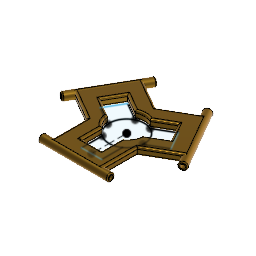
Efector Final v2 (Autodesk Fusion 360 design; units mm, degrees)
Autodesk Fusion 360 part; units mm, degrees
note: some values were not read from the file. Chosen so that the rebuilt part matches the saved one: which pieces of a blend or face edit are solid. Set by a fixed rule: which sketch regions a step uses.
sketch "Boceto1" plane through (0, 0, 0) normal (0, 0, 1) x (1, 0, 0)
  line L0 (-0.0091, 100) -> (-86.598, -50.0079)
  line L1 (-86.598, -50.0079) -> (86.6071, -49.9921)
  line L2 (86.6071, -49.9921) -> (-0.0091, 100)
  circle A0 centre (0, 0) radius 50
  line L3 (-25, 0) -> (25, 0)
  line L4 (-25, 0) -> (-24.9954, -50.0023)
  line L5 (25, 0) -> (25.0046, -49.9977)
  line L6 (12.5, -21.6506) -> (55.801, 3.3545)
  line L7 (12.5, -21.6506) -> (-12.5, 21.6506)
  line L8 (-12.5, 21.6506) -> (30.797, 46.6535)
  line L9 (12.5, 21.6506) -> (-30.8055, 46.6478)
  line L10 (12.5, 21.6506) -> (-12.5, -21.6506)
  line L11 (-12.5, -21.6506) -> (-55.8016, 3.3443)
  dimension "d3" = 50
  dimension "d4" = 50
  dimension "d6" = 360
  constraint coincident A0.centre origin
  constraint tangent L2 A0
  constraint horizontal L3
  constraint midpoint A0.centre L3
  constraint coincident L1 L4.end
  constraint perpendicular L1 L4
  constraint coincident L1 L5.end
  constraint perpendicular L1 L5
  measures "d3" distance of A0.centre L2
  measures "d4" distance of L3.start L3.end
extrude "Extruir1" add sketch "Boceto1" along normal blind 8 contours L0 A0 L9 | L2 A0 L8 | L0 A0 L11 | A0 L3 L4 L7 L8 L9 L11 | L2 A0 L6 | A0 L3 L5 L6 L8 L9 L10 | L7 L8 L9 L10 | A0 L4 L5 L6 L7 L10 L11 | L1 A0 L4 | L3 L4 L10 L11 | L3 L5 L6 L7 | L1 A0 L5 makes body 1
sketch "Boceto2" plane through (-12.498, -21.6518, 0) normal (-0.499921, -0.866071, 0) x (0.866071, -0.499921, 0)
  line L0 (-50, 0) -> (-14.4338, 0)
  line L1 (-14.4338, 0) -> (-14.4338, 8)
  line L2 (-14.4338, 8) -> (-50, 8)
  line L3 (-50, 8) -> (-50, 0)
  circle A0 centre (-50, 4) radius 2
  circle A1 centre (-50, 4) radius 4
  dimension "d9" = 4
  dimension "d10" = 8
  constraint midpoint L3 A0.centre
  constraint concentric A0 A1
  measures "d9" diameter of A0
  measures "d10" diameter of A1
extrude "Extruir2" add sketch "Boceto2" along normal blind 9.5 and the other way blind 59.5 separate body contours L3 A0 A1 | L3 A0 A1 makes body 2
sketch "Boceto3" plane through (17.2473, 29.8795, 0) normal (0.499921, 0.866071, 0) x (-0.866071, 0.499921, 0)
  circle A0 centre (50, 4) radius 2
  circle A1 centre (50, 4) radius 4
extrude "Extruir3" cut sketch "Boceto3" along normal mid plane 348 contours A0 bodies 1
sketch "Boceto4" plane through (-12.502, 21.6495, 0) normal (-0.500079, 0.86598, 0) x (-0.86598, -0.500079, 0)
  line L0 (-50, 0) -> (-14.4338, 0)
  line L1 (-14.4338, 0) -> (-14.4338, 8)
  line L2 (-14.4338, 8) -> (-50, 8)
  line L3 (-50, 8) -> (-50, 0)
  circle A0 centre (-50, 4) radius 2
  circle A1 centre (-50, 4) radius 4
  dimension "d17" = 4
  dimension "d18" = 8
  constraint midpoint L3 A0.centre
  constraint concentric A0 A1
  measures "d17" diameter of A0
  measures "d18" diameter of A1
extrude "Extruir4" add sketch "Boceto4" along normal blind 9.5 and the other way blind 59.5 separate body contours L3 A0 A1 | L3 A0 A1 makes body 3
sketch "Boceto5" plane through (-17.2527, 29.8763, 0) normal (-0.500079, 0.86598, 0) x (-0.86598, -0.500079, 0)
  circle A0 centre (-50, 4) radius 2
  circle A1 centre (-50, 4) radius 4
extrude "Extruir5" cut sketch "Boceto5" along normal mid plane 532 contours A0 bodies 1
sketch "Boceto6" plane through (-25, -0.0023, 0) normal (-1, -0.000091, 0) x (0.000091, -1, 0)
  line L0 (14.4338, 0) -> (50, 0)
  line L1 (50, 0) -> (50, 8)
  line L2 (50, 8) -> (14.4338, 8)
  line L3 (14.4338, 8) -> (14.4338, 0)
  circle A0 centre (50, 4) radius 2
  circle A1 centre (50, 4) radius 4
  dimension "d25" = 4
  dimension "d26" = 8
  constraint midpoint L1 A0.centre
  constraint concentric A0 A1
  measures "d25" diameter of A0
  measures "d26" diameter of A1
extrude "Extruir6" add sketch "Boceto6" along normal blind 9.5 and the other way blind 59.5 separate body contours L1 A0 A1 | L1 A0 A1 makes body 4
sketch "Boceto7" plane through (-34.5, -0.0032, 0) normal (-1, -0.000091, 0) x (0.000091, -1, 0)
  circle A0 centre (50, 4) radius 2
  circle A1 centre (50, 4) radius 4
extrude "Extruir7" cut sketch "Boceto7" along normal mid plane 216 contours A0 bodies 1
sketch "Boceto8" plane through (0, 0, 0) normal (0, 0, 1) x (1, 0, 0)
  circle A0 centre (0, 0) radius 17.5
  line L0 (0, 0) -> (0, -35) construction
  line L1 (10, -35) -> (10, -14.3614)
  line L2 (-10, -35) -> (-10, -14.3614)
  line L3 (-10, -35) -> (10, -35)
  line L4 (25.3109, 26.1603) -> (7.4373, 15.841)
  line L5 (35.3109, 8.8397) -> (25.3109, 26.1603)
  line L6 (35.3109, 8.8397) -> (17.4373, -1.4796)
  line L7 (-35.3109, 8.8397) -> (-17.4373, -1.4796)
  line L8 (-25.3109, 26.1603) -> (-35.3109, 8.8397)
  line L9 (-25.3109, 26.1603) -> (-7.4373, 15.841)
  dimension "d33" = 35
  dimension "d34" = 35
  dimension "d36" = 20
  dimension "d38" = 360
  constraint coincident A0.centre L0.start
  constraint vertical L0
  constraint coincident A0 L1.end
  constraint symmetric L0 L1.start L2.start
  constraint symmetric L0 L1.end L2.end
  constraint perpendicular L1 L3
  measures "d33" diameter of A0
  measures "d34" distance of A0.centre L0.end
  measures "d36" distance of L1.start L2.start
extrude "Extruir8" cut sketch "Boceto8" along normal mid plane 70 bodies 1
extrude "Extruir9" cut sketch "Boceto8" along normal blind 50 bodies 1
fillet "Empalme1" radius 2 tangency weight 2 18 edges at (40.4011, -5.5385, 8) (25.0029, -32.2146, 8) (-24.9971, -32.2192, 8) (-40.4001, -5.5459, 8) (-15.4041, 37.7577, 8) (15.3972, 37.7605, 8) (30.3109, 17.5, 8) (26.3741, 3.6801, 8) (15.1554, -8.75, 8) (10, -24.6807, 8) (0, -35, 8) (-10, -24.6807, 8) (-15.1554, -8.75, 8) (-26.3741, 3.6801, 8) (-30.3109, 17.5, 8) (-16.3741, 21.0006, 8) (0, 17.5, 8) (16.3741, 21.0006, 8) on bodies 1
fillet "Empalme2" radius 2 18 edges at (10, -24.6807, 0) (0, -35, 0) (-10, -24.6807, 0) (15.1554, -8.75, 0) (26.3741, 3.6801, 0) (30.3109, 17.5, 0) (16.3741, 21.0006, 0) (0, 17.5, 0) (-16.3741, 21.0006, 0) (-30.3109, 17.5, 0) (-26.3741, 3.6801, 0) (-15.1554, -8.75, 0) (25.0029, -32.2146, 0) (-24.9971, -32.2192, 0) (40.4011, -5.5385, 0) (15.3972, 37.7605, 0) (-15.4041, 37.7577, 0) (-40.4001, -5.5459, 0) on bodies 1
fillet "Empalme3" radius 1 1 edges at (-34.4958, -46.2738, 2.5535) on bodies 4
fillet "Empalme4" radius 1 5 edges at (-63.7807, -3.0191, 2.5535) (-29.2861, 56.7399, 5.4465) (63.7812, -3.0074, 5.4465) (29.2758, 56.7452, 2.5535) (34.5042, -46.2675, 5.4465) on bodies 2 3 4
fillet "Empalme5" radius 2 3 edges at (-29.0734, 45.648, 4) (29.065, 45.6533, 4) (54.069, 2.3543, 4) on bodies 1
